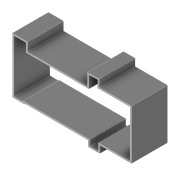
# Autodesk Inventor part: Foam_Base
Saved by Autodesk Inventor 2021 (Build 250183000, 183)
## iProperties
Created: 2021-02-18
Part Number: Foam_Base
Material: Polystyrene, Expanded
Document SubType Name: Modeling
Designer: negt20
Density: 0.05 g/cm^3
Appearance: Gray
Author: negt20
## iProperties of the stored document _3DPrint.ipt
Created: 2021-04-14
Part Number: _3DPrint
Material: Generic
Document SubType Name: Modeling
Designer: negt20
Density: 1 g/cm^3
Appearance: Default
Author: negt20
Autodesk Inventor part; units mm, degrees
ref_plane "YZ Plane" through (0, 0, 0) normal (1, 0, 0) x (0, 1, 0)
ref_plane "XZ Plane" through (0, 0, 0) normal (0, 1, 0) x (-1, 0, 0)
ref_plane "XY Plane" through (0, 0, 0) normal (0, 0, 1) x (1, 0, 0)
sketch "Sketch1" plane through (0, 0, 0) normal (0, 0, 1) x (1, 0, 0)
  line L0 (-87.5, 50) -> (87.5, 50)
  line L1 (87.5, 50) -> (87.5, -50)
  line L2 (87.5, -50) -> (-87.5, -50)
  line L3 (-87.5, -50) -> (-87.5, 50)
  point P0 (0, 0)
  point P1 (0, 50)
  point P2 (-87.5, 0)
  dimension "d0" = 175
  dimension "d1" = 100
  constraints: 8 end point, 2 midpoint, 2 parallel, 1 horizontal, 1 horizontal alignment, 1 perpendicular, 1 vertical alignment
  measures "d0" distance of L1.end L2.end
  measures "d1" distance of L0.end L1.end
extrude "Extrusion1" add sketch "Sketch1" along normal blind 25
sketch "Sketch2" plane through (0, 0, 25) normal (0, 0, 1) x (1, 0, 0)
  line L0 (-87.5, 50) -> (-87.5, -50) projected
  line L1 (-87.5, 0) -> (-62.5, 0) construction
  line L2 (87.5, 50) -> (-87.5, 50) construction
  line L3 (87.5, 50) -> (87.5, 50)
  line L4 (87.5, 50) -> (87.5, -50) construction
  line L5 (87.5, -50) -> (87.5, -50) construction
  line L6 (87.5, -50) -> (87.5, 50) construction
  line L7 (-87.5, -50) -> (87.5, -50) projected
  line L8 (87.5, 50) -> (87.5, -50)
  line L9 (-27.5, 17.5) -> (52.5, 17.5)
  line L10 (52.5, 17.5) -> (52.5, -17.5)
  line L11 (52.5, -17.5) -> (-27.5, -17.5)
  line L12 (-27.5, -17.5) -> (-27.5, 17.5)
  line L13 (-62.5, 50) -> (87.5, 50)
  line L14 (87.5, 50) -> (87.5, -50)
  line L15 (87.5, -50) -> (-62.5, -50)
  line L16 (-62.5, -50) -> (-62.5, 50)
  line L17 (-62.5, 50) -> (87.5, -50) construction
  point P0 (0, 0)
  point P1 (-27.5, 0)
  point P2 (12.5, 17.5)
  point P3 (12.5, 0)
  dimension "d4" = 25
  dimension "d5" = 80
  dimension "d6" = 35
  constraints: 30 end point, 6 equal length, 4 horizontal, 4 midpoint, 3 perpendicular, 2 point on line, 1 horizontal alignment, 1 vertical, 1 vertical alignment
  measures "d4" distance of L1.start L1.end
  measures "d5" distance of L10.end L11.end
  measures "d6" distance of L9.end L10.end
extrude "Extrusion2" [suppressed]
sketch "Sketch3" plane through (0, 0, 0) normal (0, 0, -1) x (-1, 0, 0)
  line L0 (87.5, 50) -> (87.5, -50) projected
  line L1 (87.5, 0) -> (62.5, 0)
  line L2 (62.5, 0) -> (62.5, -50) construction
  line L3 (62.5, -50) -> (-87.5, 50) construction
  line L4 (-87.5, 50) -> (-12.5, 0)
  line L5 (-12.5, 0) -> (-37.5, 0) construction
  line L6 (-37.5, 0) -> (-37.5, -16.5)
  line L7 (-37.5, -16.5) -> (-15.5, -16.5)
  line L8 (-15.5, -16.5) -> (-15.5, -21.5)
  line L9 (-15.5, -21.5) -> (-9.5, -21.5)
  line L10 (-9.5, -21.5) -> (-9.5, -17.5)
  line L11 (-9.5, -17.5) -> (36.5, -17.5)
  line L12 (43, 0) -> (43, 18.5)
  line L13 (43, 18.5) -> (34.5, 18.5)
  line L14 (34.5, 18.5) -> (34.5, 12.4958)
  line L15 (36.5, -17.5) -> (36.5, -18)
  line L16 (36.5, -18) -> (43, -18)
  line L17 (43, -18) -> (43, 0)
  line L18 (34.5, 12.4958) -> (-9, 12.4958)
  line L19 (-9, 12.4958) -> (-9, 20.9958)
  line L20 (-9, 20.9958) -> (-15, 20.9958)
  line L21 (-15, 20.9958) -> (-15, 16)
  line L22 (-15, 16) -> (-37.5, 16)
  line L23 (-37.5, 16) -> (-37.5, 0)
  line L24 (-15, 16) -> (-15.5, -16.5) construction
  line L25 (-9.5, -17.5) -> (-9, 12.4958) construction
  point P0 (0, 0)
  dimension "d9" = 25
  dimension "d10" = 25
  dimension "d11" = 16.5
  dimension "d12" = 22
  dimension "d13" = 5
  dimension "d14" = 6
  dimension "d15" = 4
  dimension "d16" = 46
  dimension "d18" = 18.5
  dimension "d20" = 0.5
  dimension "d21" = 6.5
  dimension "d22" = 18
  dimension "d23" = 8.5
  dimension "d25" = 8.5
  dimension "d26" = 6
  dimension "d28" = 22.5
  dimension "d29" = 50
  dimension "d34" = 16
  dimension "d35" = 30
  constraints: 50 end point, 11 perpendicular, 4 horizontal, 4 vertical, 2 midpoint, 1 coincident, 1 collinear, 1 parallel
  measures "d9" distance of L1.start L1.end
  measures "d10" distance of L5.start L5.end
  measures "d11" distance of L5.end L6.end
  measures "d12" distance of L6.end L7.end
  measures "d13" distance of L7.end L8.end
  measures "d14" distance of L8.end L9.end
  measures "d15" distance of L9.end L10.end
  measures "d16" distance of L10.end L11.end
  measures "d18" distance of L12.start L12.end
  measures "d20" distance of L11.end L15.end
  measures "d21" distance of L15.end L16.end
  measures "d22" distance of L16.end L12.start
  measures "d23" distance of L12.end L13.end
  measures "d25" distance of L18.end L19.end
  measures "d26" distance of L19.end L20.end
  measures "d28" distance of L21.end L22.end
  measures "d29" distance of L1.end L2.end
  measures "d34" distance of L22.end L5.end
  measures "d35" distance of L10.end L18.end
extrude "Extrusion3" cut sketch "Sketch3" against normal blind 25
shell "Shell1" thickness 1 removed faces 6 at (3, 40.3319, 0) at (-87.5, 16.6667, 8.3333) at (29.1667, 50, 8.3333) at (87.5, -16.6667, 8.3333) at (-29.1667, -50, 8.3333) at (3, 40.3319, 25)
body "Solid1"
